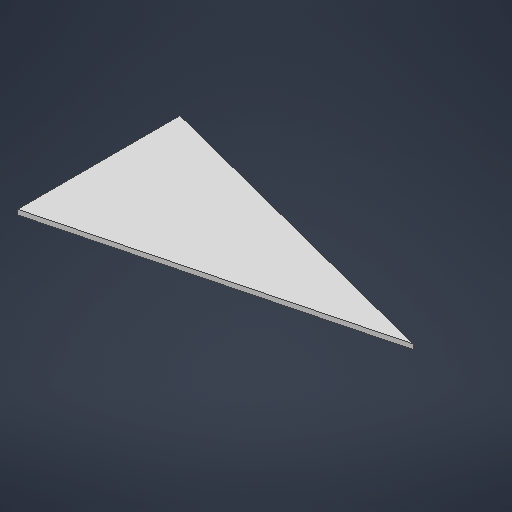
# Autodesk Inventor part: Pieza3
Saved by Autodesk Inventor 2027 (Build 310192060, 192F)
## iProperties
Created: 2026-08-23
Part Number: Pieza3
Material: Genérico
Document SubType Name: Modeling
Designer: Leandro
Density: 1 g/cm^3
Appearance: Valor por defecto
Author: Leandro
Autodesk Inventor part; units mm, degrees
ref_plane "YZ Plane" through (0, 0, 0) normal (1, 0, 0) x (0, 1, 0)
ref_plane "XZ Plane" through (0, 0, 0) normal (0, 1, 0) x (-1, 0, 0)
ref_plane "XY Plane" through (0, 0, 0) normal (0, 0, 1) x (1, 0, 0)
sketch "Boceto1" plane through (0, 0, 0) normal (0, 1, 0) x (-1, 0, 0)
  line L0 (0, -1.7078) -> (0, -101.7078)
  line L1 (0, -101.7078) -> (-193.6492, -51.7078)
  line L2 (-193.6492, -51.7078) -> (0, -1.7078)
  point P0 (0, 0)
  dimension "d0" = 100
  dimension "d1" = 200
  constraints: 6 end point, 1 vertical
  measures "d0" distance of L0.start L0.end
  measures "d1" distance of L0.end L1.end
extrude "Extrusión1" add sketch "Boceto1" along normal mid plane 3
